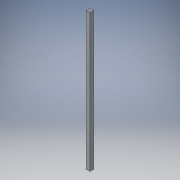
# Autodesk Inventor part: AXp12s
Saved by Autodesk Inventor 2019.3 (Build 233278000, 278)
## iProperties
Company: Unknown
Created: 2018-11-05
Part Number: AXp12s
Material: Generic
Description: Unknown
Document SubType Name: Modeling
Designer: Varga Daniel
Density: 1 g/cm^3
Appearance: Default
Axle_hole_fillet: 0,300 mm
Title: Axeis 5s
Author: Unknown
Autodesk Inventor part; units mm, degrees
ref_plane "YZ Plane" through (0, 0, 0) normal (1, 0, 0) x (0, 1, 0)
ref_plane "XZ Plane" through (0, 0, 0) normal (0, 1, 0) x (-1, 0, 0)
ref_plane "XY Plane" through (0, 0, 0) normal (0, 0, 1) x (1, 0, 0)
derived "One_sided_axle_base.ipt"
derived "Base_part.ipt"
sketch "Axle_hole_sketch" plane through (0, 0, 0) normal (0, 1, 0) x (-1, 0, 0)
  line L0 (-14.3207, 2.4447) -> (-17.4707, 2.4447)
  line L1 (-17.7707, 2.7447) -> (-17.7707, 5.8947)
  line L2 (-17.4707, 6.1947) -> (-14.3207, 6.1947)
  line L3 (-14.0207, 5.8947) -> (-14.0207, 2.7447)
  line L4 (-14.0207, 2.4447) -> (-17.7707, 6.1947) construction
  line L5 (-17.7707, 2.4447) -> (-14.0207, 6.1947) construction
  arc A0 (-14.3207, 2.4447) -> (-14.0207, 2.7447) centre (-14.3207, 2.7447) ccw
  arc A1 (-17.7707, 2.7447) -> (-17.4707, 2.4447) centre (-17.4707, 2.7447) ccw
  arc A2 (-17.4707, 6.1947) -> (-17.7707, 5.8947) centre (-17.4707, 5.8947) ccw
  arc A3 (-14.0207, 5.8947) -> (-14.3207, 6.1947) centre (-14.3207, 5.8947) ccw
  point P0 (0, 0)
  point P1 (-15.8957, 4.3197)
sketch "Sketch3" plane through (0, 0, 0) normal (0, 1, 0) x (-1, 0, 0)
  line L0 (-14.0207, 5.8947) -> (-14.0207, 2.7447) construction
  arc A0 (-14.3207, 2.4447) -> (-14.0207, 2.7447) centre (-14.3207, 2.7447) ccw construction
  line L1 (-14.3207, 2.4447) -> (-17.4707, 2.4447) construction
  arc A1 (-17.7707, 2.7447) -> (-17.4707, 2.4447) centre (-17.4707, 2.7447) ccw construction
  line L2 (-17.7707, 2.7447) -> (-17.7707, 5.8947) construction
  arc A2 (-17.4707, 6.1947) -> (-17.7707, 5.8947) centre (-17.4707, 5.8947) ccw construction
  line L3 (-17.4707, 6.1947) -> (-14.3207, 6.1947) construction
  arc A3 (-14.0207, 5.8947) -> (-14.3207, 6.1947) centre (-14.3207, 5.8947) ccw construction
  line L4 (1.575, 1.875) -> (-1.575, 1.875)
  line L5 (-1.875, 1.575) -> (-1.875, -1.575)
  line L6 (-1.575, -1.875) -> (1.575, -1.875)
  line L7 (1.875, -1.575) -> (1.875, 1.575)
  line L8 (1.875, 1.875) -> (-1.875, -1.875) construction
  line L9 (-1.875, 1.875) -> (1.875, -1.875) construction
  arc A4 (1.875, 1.575) -> (1.575, 1.875) centre (1.575, 1.575) ccw
  arc A5 (-1.575, 1.875) -> (-1.875, 1.575) centre (-1.575, 1.575) ccw
  arc A6 (-1.875, -1.575) -> (-1.575, -1.875) centre (-1.575, -1.575) ccw
  arc A7 (1.575, -1.875) -> (1.875, -1.575) centre (1.575, -1.575) ccw
  point P0 (0, 0)
  point P1 (0, 0)
  point P2 (0, 0)
  dimension "d9" = 3.75
  dimension "d10" = 0.3
  dimension "d11" = 3.75
  dimension "d12" = 3.75
  dimension "d13" = 0.3
  constraints: 12 end point, 8 point on circle, 8 point on line, 8 tangent, 4 centre point, 3 equal radius, 3 midpoint, 2 parallel, 1 coincident, 1 horizontal, 1 perpendicular
  measures "d9" distance between parallel lines of L3 L1
  measures "d10" radius of A0
  measures "d11" distance between parallel lines of L6 L4
  measures "d12" distance between parallel lines of L7 L5
  measures "d13" radius of A4
extrude "Extrusion2" add sketch "Sketch3" along normal blind 120
fillet "Fillet2" radius 0.4 16 edges at (1.7871, 120, 1.7871) (1.875, 120, 0) (1.7871, 120, -1.7871) (0, 120, -1.875) (-1.7871, 120, -1.7871) (-1.875, 120, 0) (-1.7871, 120, 1.7871) (0, 120, 1.875) (1.7871, 0, 1.7871) (1.875, 0, 0) (1.7871, 0, -1.7871) (0, 0, -1.875) (-1.7871, 0, -1.7871) (-1.875, 0, 0) (-1.7871, 0, 1.7871) (0, 0, 1.875)
equation "\"d11\" = d9"
equation "\"d12\" = d11"
equation "\"d13\" = d10"
equation "\"d14\" = Straigh_axle_length"
equation "\"d16\" = Upper_fillet"
equation "\"Straigh_axle_length\" = 120"
equation "\"Upper_fillet\" = 0.4"
body "Solid1"
